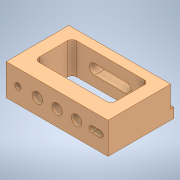
# Autodesk Inventor part: ASF-10003
Saved by Autodesk Inventor 2020 (Build 240168000, 168)
## iProperties
Created: 2014-09-24
Part Number: ASF-10003
Material: Generic
Document SubType Name: Modeling
Designer: map
Density: 1 g/cm^3
Appearance: Default
Mass: 27.2429 g
Surface Area: 107.547 cm^2
Volume: 27.2429 cm^3
Description: Aperture mount with slot
Sending System: SolidWorks 2015
Last Author: ml2377
Last Saved: 2016-05-27
Author: map
Autodesk Inventor part; units mm, degrees
ref_plane "XZ Plane" through (0, 0, 0) normal (0, 1, 0) x (-1, 0, 0)
ref_plane "XY Plane" through (0, 0, 0) normal (0, 0, 1) x (1, 0, 0)
ref_plane "Work Plane1" through (-32.5, 0, 0) normal (1, 0, 0) x (0, 1, 0)
sketch "Sketch1" plane through (-32.5, 0, 0) normal (1, 0, 0) x (0, 1, 0)
  line L0 (-21, 10) -> (-21, -10)
  line L1 (19, -3.75) -> (21, -3.75)
  line L2 (21, -10) -> (-21, -10)
  line L3 (19, 10) -> (19, -3.75)
  line L4 (19, 10) -> (-21, 10)
  line L5 (21, -3.75) -> (21, -10)
  constraints: 12 end point, 4 vertical, 2 horizontal
extrude "Extrusion4" add sketch "Sketch1" along normal blind 65
sketch "Sketch2" plane through (-32.5, -21, 10) normal (0, 0, 1) x (1, 0, 0)
  line L0 (57, 10) -> (57, 34)
  line L1 (57, 34) -> (8, 34)
  line L2 (8, 34) -> (8, 10)
  line L3 (8, 10) -> (57, 10)
  constraints: 8 end point, 2 horizontal, 2 vertical
extrude "Extrusion3" cut sketch "Sketch2" against normal blind 20
sketch "Sketch3" plane through (-32.5, 19, 10) normal (0, 1, 0) x (1, 0, 0)
  line L0 (42.5, 13.3) -> (22.5, 13.3)
  arc A0 (22.5, 13.3) -> (22.5, 6.7) centre (22.5, 10) ccw
  arc A1 (42.5, 6.7) -> (42.5, 13.3) centre (42.5, 10) ccw
  line L1 (22.5, 6.7) -> (42.5, 6.7)
  constraints: 4 end point, 4 point on circle, 2 centre point, 2 horizontal, 1 equal radius, 1 parallel
extrude "Extrusion2" cut sketch "Sketch3" against normal blind 6
fillet "Fillet4" radius 3 1 edges at (24.5, 13, 0)
fillet "Fillet3" radius 3 1 edges at (24.5, -11, 0)
fillet "Fillet2" radius 3 1 edges at (-24.5, -11, 0)
fillet "Fillet1" radius 3 1 edges at (-24.5, 13, 0)
sketch "Sketch7" plane through (-32.5, -21, -10) normal (0, -1, 0) x (1, 0, 0)
  line L0 (45, 10) -> (20, 10)
  line L1 (11, 20) -> (54, 20) construction
  line L2 (32.5, 20) -> (32.5, 0) construction
  line L3 (0, 0) -> (65, 0) construction
  point P0 (32.5, 10)
  point P1 (32.5, 10)
  dimension "d41" = 25
  constraints: 4 end point, 4 midpoint, 1 coincident, 1 horizontal
  measures "d41" distance of L0.start L0.end
hole "M6CLR" at (0, -21, 0) at (-12.5, -21, 0) at (12.5, -21, 0) direction (0, 1, 0) diameter 6.6 depth 10 clearance for "Countersunk Flat Head Screw ISO 2009/7046" size "M6" standard "ISO"
sketch "Sketch5" plane through (-32.5, -21, -10) normal (0, -1, 0) x (1, 0, 0)
  point P0 (7.5, 10)
hole "4H7" at (-25, -21, 0) direction (0, 1, 0) diameter 4 depth 9 tip angle 118
sketch "Sketch4" plane through (-32.5, -21, -10) normal (0, -1, 0) x (1, 0, 0)
  arc A0 (60, 8) -> (60, 12) centre (60, 10) ccw
  line L0 (55, 8) -> (60, 8)
  line L1 (60, 12) -> (55, 12)
  arc A1 (55, 12) -> (55, 8) centre (55, 10) ccw
  dimension "d42" = 4
  dimension "d43" = 5
  constraints: 4 end point, 4 point on circle, 2 centre point, 2 horizontal, 1 equal radius, 1 parallel
  measures "d42" distance between parallel lines of L0 L1
  measures "d43" distance of A0.centre A1.centre
extrude "Extrusion1" cut sketch "Sketch4" against normal blind 9
body "Solid3"
